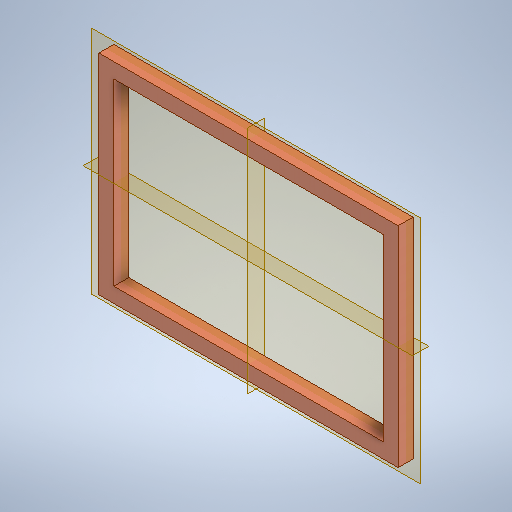
# Autodesk Inventor part: Mesa_001
Saved by Autodesk Inventor 2025.2 (Build 292293000, 293)
## iProperties
Created: 2025-04-07
Part Number: Mesa_001
Material: Madeira (Nogueira)
Document SubType Name: Modeling
Designer: Formação
Density: 0.55 g/cm^3
Appearance: Nogueira - Natural polido
Author: Formação
Autodesk Inventor part; units mm, degrees
sketch "Esboço1" plane through (0, 0, 0) normal (0, 0, 1) x (1, 0, 0)
  line L0 (-2500, 1750) -> (2500, 1750)
  line L1 (2500, 1750) -> (2500, -1750)
  line L2 (2500, -1750) -> (-2500, -1750)
  line L3 (-2500, -1750) -> (-2500, 1750)
  line L4 (-2500, 1750) -> (2500, -1750) construction
  line L5 (2500, 1750) -> (-2500, -1750) construction
  line L6 (-2250, 1500) -> (2250, 1500)
  line L7 (2250, 1500) -> (2250, -1500)
  line L8 (2250, -1500) -> (-2250, -1500)
  line L9 (-2250, -1500) -> (-2250, 1500)
  line L10 (-2250, 1500) -> (2250, -1500) construction
  line L11 (2250, 1500) -> (-2250, -1500) construction
  point P0 (0, 0)
  point P1 (0, 0)
  point P2 (0, 0)
  dimension "d0" = 5000
  dimension "d1" = 3500
  dimension "d2" = 250
  dimension "d3" = 250
  constraints: 24 end point, 5 midpoint, 4 parallel, 3 coincident, 2 horizontal, 2 perpendicular
  measures "d0" distance of L0.end L0.start
  measures "d1" distance of L1.end L0.end
  measures "d2" distance between parallel lines of L0 L6
  measures "d3" distance between parallel lines of L1 L7
extrude "Extrusão1" add sketch "Esboço1" along normal mid plane 250
